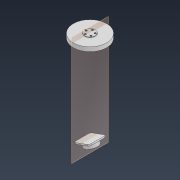
# Autodesk Inventor part: CH_01_0044_motor_end
Saved by Autodesk Inventor 2022 (Build 260153000, 153)
## iProperties
Created: 2022-08-11
Part Number: CH_01_0044_motor_end
Material: Generic
Document SubType Name: Modeling
Designer: Tomasz Krakowski
Density: 1 g/cm^3
Appearance: Default
Author: Tomasz Krakowski
Autodesk Inventor part; units mm, degrees
ref_plane "XZ Plane" through (0, 0, 0) normal (0, 1, 0) x (-1, 0, 0)
ref_plane "XY Plane" through (0, 0, 0) normal (0, 0, 1) x (1, 0, 0)
sketch "Sketch1" plane through (0, 0, 0) normal (0, 1, 0) x (-1, 0, 0)
  circle A0 centre (0, 0) radius 12.5
  dimension "d0" = 25
  constraints: 1 centre point, 1 coincident
  measures "d0" diameter of A0
extrude "Extrusion1" add sketch "Sketch1" along normal blind 0.9
sketch "Sketch2" plane through (0, 0, 0) normal (0, -1, 0) x (1, 0, 0)
  circle A0 centre (0, 0) radius 39.6
  dimension "d3" = 79.2
  constraints: 1 centre point, 1 coincident
  measures "d3" diameter of A0
extrude "Extrusion2" add sketch "Sketch2" along normal blind 10
sketch "Sketch3" plane through (0, 0.9, 0) normal (0, 1, 0) x (1, 0, 0)
  line L0 (0, 0) -> (-9, 0) construction
  circle A0 centre (0, 0) radius 9 construction
  point P0 (-2.7812, -8.5595)
  point P1 (7.2812, -5.2901)
  point P2 (7.2812, 5.2901)
  point P3 (-2.7812, 8.5595)
  point P4 (-2.7812, 8.5595)
  point P5 (7.2812, 5.2901)
  point P6 (7.2812, -5.2901)
  point P7 (-2.7812, -8.5595)
  dimension "d6" = 18
  dimension "d9" = 360
  constraints: 7 coincident, 2 end point, 1 horizontal, 1 horizontal alignment, 8 other
hole "Hole2" at (-9, 0.9, 0) at (-2.7812, 0.9, -8.5595) at (7.2812, 0.9, -5.2901) at (7.2812, 0.9, 5.2901) at (-2.7812, 0.9, 8.5595) direction (0, -1, 0) diameter 3.242 end through all countersink diameter 4 countersink angle 90 thread size "M4x0.7" class "6H" standard "ISO Metric profile"
sketch "Sketch4" plane through (0, 0, 0) normal (0, 0, 1) x (1, 0, 0)
  line L0 (18.2808, -210.8501) -> (-19.3069, -224.5309)
  line L1 (-19.3069, -224.5309) -> (-18.2808, -227.3499)
  line L2 (-18.2808, -227.3499) -> (19.3069, -213.6691)
  line L3 (19.3069, -213.6691) -> (18.2808, -210.8501)
  line L4 (18.2808, -210.8501) -> (-18.2808, -227.3499) construction
  line L5 (-19.3069, -224.5309) -> (19.3069, -213.6691) construction
  line L6 (12.5, 0.9) -> (-12.5, 0.9) construction
  line L7 (0, 0.9) -> (0, -219.1) construction
  point P0 (0, 0)
  dimension "d25" = 40
  dimension "d27" = 3
  dimension "d28" = 70
  dimension "d29" = 220
  constraints: 14 end point, 3 midpoint, 2 parallel, 1 perpendicular, 1 vertical
  measures "d25" distance of L1.end L2.end
  measures "d27" distance of L2.end L0.start
  measures "d28" angle of L7 L0
  measures "d29" distance from line of L7.end L6
extrude "Extrusion3" add sketch "Sketch4" along normal mid plane 40
sketch "Sketch5" plane through (19.3069, -213.6691, -20) normal (0.3420201, -0.9396926, 0) x (0.9396926, 0.3420201, 0)
  line L0 (0, 0) -> (0, 40) projected
  line L1 (0, 20) -> (-20, 20) construction
  line L2 (-20, 20) -> (-20, 0) construction
  line L3 (0, 0) -> (-40, 0) projected
  circle A0 centre (-20, 20) radius 15
  point P0 (54.9366, 20)
  dimension "d32" = 30
  constraints: 4 end point, 2 midpoint, 2 perpendicular, 1 centre point, 1 coincident
  measures "d32" diameter of A0
extrude "Extrusion4" add sketch "Sketch5" along normal blind 10
fillet "Fillet1" radius 5 4 edges at (18.7939, -212.2596, 20) (-18.7939, -225.9404, 20) (18.7939, -212.2596, -20) (-18.7939, -225.9404, -20)
body "Solid1"
